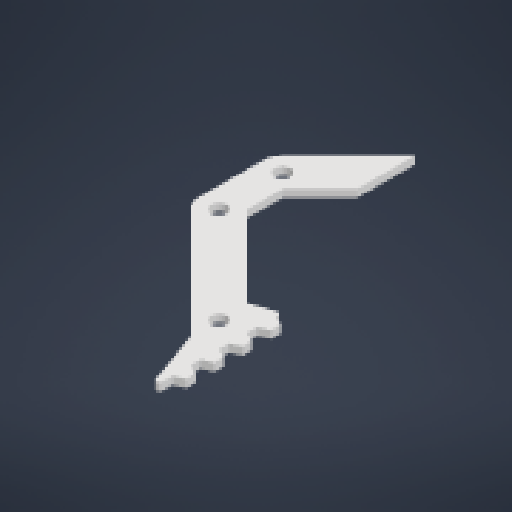
# Autodesk Inventor part: claw_dynamic_gripper
Saved by Autodesk Inventor 2026 (Build 300175000, 175)
## iProperties
Created: 2025-03-27
Part Number: claw_dynamic_gripper
Material: Generic
Document SubType Name: Modeling
Designer: paris
Density: 1 g/cm^3
Appearance: Default
Author: paris
Autodesk Inventor part; units mm, degrees
ref_plane "YZ Plane" through (0, 0, 0) normal (1, 0, 0) x (0, 1, 0)
ref_plane "XZ Plane" through (0, 0, 0) normal (0, 1, 0) x (-1, 0, 0)
ref_plane "XY Plane" through (0, 0, 0) normal (0, 0, 1) x (1, 0, 0)
sketch "Sketch1" plane through (0, 0, 0) normal (0, 1, 0) x (-1, 0, 0)
  line L0 (0, 0) -> (0, -30)
  line L1 (0, 0) -> (0.75, 0) construction
  arc A0 (1.4548, 0.2565) -> (0, 0) centre (0.75, 0) ccw
  line L2 (1.4548, 0.2565) -> (6.5322, -13.6936)
  line L3 (0, -30) -> (0.75, -30) construction
  circle A1 centre (0.75, -30) radius 0.75
  line L4 (1.0065, -30.7048) -> (6.5322, -28.6936)
  line L5 (6.5322, -13.6936) -> (6.5322, -28.6936) construction
  line L6 (6.5322, -13.6936) -> (35.2454, -42.4068)
  line L7 (6.5322, -13.6936) -> (66.5322, -13.6936) construction
  line L8 (6.5322, -28.6936) -> (27.7454, -49.9068)
  line L9 (6.5322, -28.6936) -> (36.5322, -28.6936) construction
  line L10 (27.7454, -49.9068) -> (27.7454, -58.9068)
  line L11 (27.7454, -58.9068) -> (6.5322, -80.12)
  line L12 (27.7454, -58.9068) -> (57.7454, -58.9068) construction
  line L13 (35.2454, -42.4068) -> (27.7454, -49.9068) construction
  arc A2 (36.7987, -46.1568) -> (35.2454, -42.4068) centre (31.4954, -46.1568) ccw
  line L14 (36.7987, -46.1568) -> (36.7987, -62.6568)
  line L15 (27.7454, -58.9068) -> (27.7454, -73.9068) construction
  line L16 (27.7454, -73.9068) -> (16.5322, -85.12)
  line L17 (27.7454, -73.9068) -> (35.2454, -66.4068)
  line L18 (27.7454, -58.9068) -> (35.2454, -66.4068) construction
  arc A3 (35.2454, -66.4068) -> (36.7987, -62.6568) centre (31.4954, -62.6568) ccw
  line L19 (6.5322, -80.12) -> (16.5322, -80.12) construction
  line L20 (16.5322, -80.12) -> (16.5322, -85.12) construction
  line L21 (16.5322, -110.12) -> (6.5322, -110.12)
  line L22 (6.5322, -110.12) -> (6.5322, -80.12)
  line L23 (16.5322, -85.12) -> (16.5322, -110.12)
  circle A4 centre (11.5322, -87.62) radius 2
  circle A5 centre (11.5322, -102.62) radius 2
  line L24 (0, -3.6658) -> (-2.5, -3.6658)
  line L25 (-2.5, -3.6658) -> (-2.5, -6.1658)
  line L26 (-2.5, -6.1658) -> (0, -6.1658)
  line L27 (0, -6.1658) -> (0, -3.6658)
  line L28 (-2.5, -3.6658) -> (0, -2.5)
  line L29 (-2.5, -6.1658) -> (0, -7.3315)
  line L30 (0, -10.9973) -> (-2.5, -10.9973)
  line L31 (-2.5, -10.9973) -> (-2.5, -13.4973)
  line L32 (-2.5, -13.4973) -> (0, -13.4973)
  line L33 (-2.5, -10.9973) -> (0, -9.8315)
  line L34 (-2.5, -13.4973) -> (0, -14.6631)
  line L35 (-2.5, -18.3288) -> (-2.5, -20.8288)
  line L36 (-2.5, -20.8288) -> (0, -21.9946)
  line L37 (-2.5, -20.8288) -> (0, -20.8288)
  line L38 (0, -18.3288) -> (-2.5, -18.3288)
  line L39 (-2.5, -18.3288) -> (0, -17.1631)
  line L40 (-2.5, -25.6604) -> (0, -24.4946)
  line L41 (0, -25.6604) -> (-2.5, -25.6604)
  line L42 (-2.5, -25.6604) -> (-2.5, -28.1604)
  line L43 (-2.5, -28.1604) -> (0, -28.1604)
  line L44 (-2.5, -28.1604) -> (0, -29.3262)
  circle A6 centre (6.5322, -21.1936) radius 2
  circle A7 centre (31.4954, -46.1568) radius 2
  circle A8 centre (31.4954, -62.6568) radius 2
  line L45 (18.0663, -78.6361) -> (18.0663, -68.0295) projected
  line L46 (20.5412, -81.111) -> (18.0663, -78.6361) projected
  line L47 (38.2189, -63.4333) -> (20.5412, -81.111) projected
  line L48 (38.2189, -63.4333) -> (30.4407, -55.6551) projected
  line L49 (18.0663, -68.0295) -> (30.4407, -55.6551) projected
  line L50 (18.0663, -78.6361) -> (18.0663, -83.5859)
  point P0 (18.0663, -68.5859)
  dimension "d2" = 30
  dimension "d17" = 0.75
  dimension "d18" = 20
  dimension "d19" = 0.75
  dimension "d20" = 70
  dimension "d21" = 15
  dimension "d28" = 45
  dimension "d29" = 30
  dimension "d30" = 45
  dimension "d31" = 9
  dimension "d34" = 135
  dimension "d35" = 15
  dimension "d36" = 135
  dimension "d38" = 10
  dimension "d39" = 30
  dimension "d40" = 30
  dimension "d41" = 7.5
  dimension "d42" = 5
  dimension "d43" = 7.5
  dimension "d44" = 5
  dimension "d45" = 4
  dimension "d46" = 4
  dimension "d47" = 2.5
  dimension "d48" = 2.5
  dimension "d49" = 25
  dimension "d50" = 25
  dimension "d51" = 2.5
  dimension "d52" = 2.5
  dimension "d53" = 2.5
  dimension "d54" = 25
  dimension "d55" = 25
  dimension "d56" = 2.5
  dimension "d57" = 2.5
  dimension "d58" = 2.5
  dimension "d59" = 25
  dimension "d60" = 25
  dimension "d61" = 2.5
  dimension "d62" = 2.5
  dimension "d63" = 2.5
  dimension "d64" = 25
  dimension "d65" = 25
  dimension "d66" = 2.5
  dimension "d69" = 4
  dimension "d70" = 4
  dimension "d71" = 4
  constraints: 90 end point, 11 horizontal, 9 centre point, 9 parallel, 8 perpendicular, 8 point on circle, 6 coincident, 5 vertical, 3 midpoint, 3 tangent, 2 equal length, 1 point on line, 18 other
  measures "d2" distance of L1.start L3.start
  measures "d17" distance of L1.start L1.end
  measures "d18" angle to the sketch y axis of L2
  measures "d19" distance of L3.start L3.end
  measures "d20" angle to the sketch y axis of L4
  measures "d21" distance of L4.end L2.end
  measures "d28" angle of L6 L7
  measures "d29" distance of L8.end L4.end
  measures "d30" angle of L8 L9
  measures "d31" distance of L8.end L10.end
  measures "d34" angle of L11 L12
  measures "d35" distance of L10.end L15.end
  measures "d36" angle of L15 L16
  measures "d38" distance of L21.start L21.end
  measures "d39" distance of L19.end L21.start
  measures "d40" distance of L10.end L11.end
  measures "d41" distance from line of L21 point (11.532, -102.62)
  measures "d42" distance from line of L22 point (11.532, -102.62)
  measures "d43" vertical distance of L11.end point (11.532, -87.62)
  measures "d44" distance from line of L22 point (11.532, -87.62)
  measures "d45" diameter of A4
  measures "d46" diameter of A5
  measures "d47" distance of L26.end L25.end
  measures "d48" distance of L25.end L24.end
  measures "d49" angle of L26 L29
  measures "d50" angle of L24 L28
  measures "d51" distance of L1.start L28.end
  measures "d52" distance of L32.end L31.end
  measures "d53" distance of L31.end L31.start
  measures "d54" angle of L32 L34
  measures "d55" angle of L30 L33
  measures "d56" distance of L33.end L29.end
  measures "d57" distance of L37.end L35.end
  measures "d58" distance of L35.end L39.start
  measures "d59" angle of L37 L36
  measures "d60" angle of L38 L39
  measures "d61" distance of L39.end L34.end
  measures "d62" distance of L43.end L42.end
  measures "d63" distance of L42.end L40.start
  measures "d64" angle of L43 L44
  measures "d65" angle of L41 L40
  measures "d66" distance of L40.end L36.end
  measures "d69" diameter of A6
  measures "d70" diameter of A7
  measures "d71" diameter of A8
extrude "Extrusion2" add sketch "Sketch1" along normal blind 2 contours A0 L2 L6 A2 L14 L48 L49 L10 L8 L4 A1 L0 | L0 L24 L28 | L0 L26 L25 L24 | L0 L29 L26 | L0 L30 L33 | L14 A3 L17 L16 L46 L45 L11 L10 L49 L48 | L0 L32 L31 L30 | L0 L34 L32 | L0 L38 L39 | L16 L50 L46 | L0 L37 L35 L38 | A1 | L0 L36 L37 | L44 L43 L0 | L0 L41 L40 | L43 L42 L41 L0
body "Solid2"
